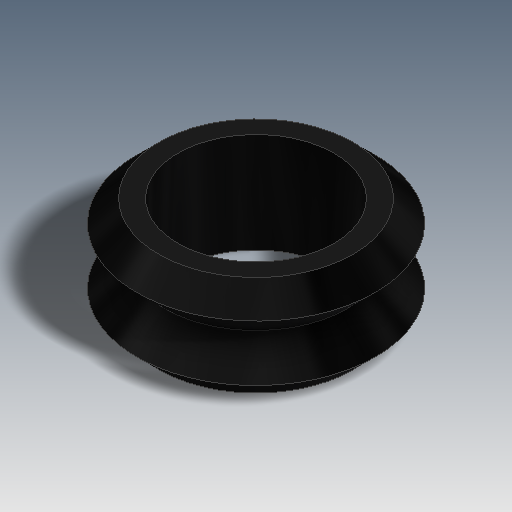
# Autodesk Inventor part: Delrin V-Wheel
Saved by Autodesk Inventor 2020 (Build 240168000, 168)
## iProperties
Created: 2016-04-09
Part Number: Delrin V-Wheel
Material: Generic
Document SubType Name: Modeling
Designer: Ben
Density: 1 g/cm^3
Appearance: Default
Author: Ben
Autodesk Inventor part; units mm, degrees
ref_plane "YZ Plane" through (0, 0, 0) normal (1, 0, 0) x (0, 1, 0)
ref_plane "XZ Plane" through (0, 0, 0) normal (0, 1, 0) x (-1, 0, 0)
ref_plane "XY Plane" through (0, 0, 0) normal (0, 0, 1) x (1, 0, 0)
sketch "Sketch1" plane through (0, 0, 0) normal (0, 0, 1) x (1, 0, 0)
  line L0 (0, 0) -> (0, 12.4297) construction
  line L1 (7.987, 0) -> (9.9363, 0)
  line L2 (9.9363, 0) -> (12.195, 2.2587)
  line L3 (12.195, 2.2587) -> (9.3387, 5.115)
  line L4 (9.3387, 5.115) -> (12.195, 7.9713)
  line L5 (12.195, 7.9713) -> (9.9363, 10.23)
  line L6 (9.9363, 10.23) -> (7.987, 10.23)
  line L7 (7.987, 10.23) -> (7.987, 0)
  line L8 (7.987, 5.115) -> (38.026, 5.115) construction
  line L9 (0, 0) -> (31.3179, 0) construction
  dimension "d0" = 10.23
  dimension "d1" = 15.974
  dimension "d2" = 90
  dimension "d4" = 90
  dimension "d5" = 24.39
  constraints: 20 end point, 4 perpendicular, 1 collinear, 1 midpoint, 1 parallel, 1 point on line, 1 vertical, 1 other
  measures "d0" distance of L6.end L1.start
  measures "d1" diameter of L7 L0
  measures "d2" angle of L2 L5
  measures "d4" angle of L3 L4
  measures "d5" diameter of L4.end L0
revolve "Revolution1" add sketch "Sketch1" angle 360 about axis through (0, 0, 0) along (0, 1, 0)
body "Solid1"
